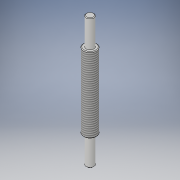
# Autodesk Inventor part: Вал
Saved by Autodesk Inventor 2019 (Build 230136000, 136)
## iProperties
Created: 2021-03-17
Part Number: Вал
Material: Типовые
Document SubType Name: Modeling
Designer: Петров Иван
Density: 1 g/cm^3
Appearance: По умолчанию
Author: Петров Иван
Autodesk Inventor part; units mm, degrees
ref_plane "YZ Plane" through (0, 0, 0) normal (1, 0, 0) x (0, 1, 0)
sketch "Sketch1" plane through (0, 0, 0) normal (0, 1, 0) x (-1, 0, 0)
  circle A0 centre (0, 0) radius 3
  dimension "d0" = 6
  constraints: 1 centre point, 1 coincident
  measures "d0" diameter of A0
extrude "Extrusion1" add sketch "Sketch1" along normal blind 100
chamfer "Chamfer1" distance 0.5 angle 45 2 edges at (3, 100, 0) (3, 0, 0)
ref_plane "Work Plane1" through (25.9576, 21.0507, -5.9332) normal (0, 1, 0) x (0.930981, 0, 0.3650675)
sketch "Sketch2" plane through (25.9576, 21.0507, -5.9332) normal (0, 1, 0) x (0.930981, 0, 0.3650675)
  circle A0 centre (-22, -15) radius 3 projected
  circle A1 centre (-22, -15) radius 5
  point P0 (-22, -15)
  dimension "d8" = 10
  constraints: 1 centre point, 1 coincident
  measures "d8" diameter of A1
ref_plane "Work Plane2" through (-26.6757, 78.9493, -24.1044) normal (0, -1, 0) x (0.930981, 0, 0.3650675)
extrude "Extrusion2" add sketch "Sketch2" along normal up to surface (57.8986 mm away)
chamfer "Chamfer2" distance 0.5 angle 45 2 edges at (-4.6549, 78.9493, -1.8253) (-4.6549, 21.0507, -1.8253)
thread "Thread2" size "M10x1.5" class "6g" standard "ANSI Metric M Profile" full length
body "Solid1"
